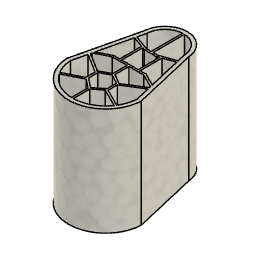
Molde fijo (Autodesk Fusion 360 design; units mm, degrees)
Autodesk Fusion 360 part; units mm, degrees
note: some values were not read from the file. Set by a fixed rule: which sketch regions a step uses.
sketch "Boceto1" plane through (0, 0, 0) normal (0, 0, 1) x (1, 0, 0)
  line L0 (0, -31.5) -> (3, -31.5) construction
  circle A0 centre (3, -22.5) radius 1.5 construction
  circle A1 centre (3, -10.5) radius 1.5 construction
  circle A2 centre (-5.5, -17.5) radius 1.5 construction
  line L1 (0, -35) -> (0, -31.5) construction
  line L2 (0, -35) -> (0, -5) construction
  line L3 (0, -20) -> (7.4517, -20) construction
  circle A3 centre (0, -16.5) radius 1.5 construction
  circle A4 centre (5.5, -17.5) radius 1.5 construction
  circle A5 centre (-3, -22.5) radius 1.5 construction
  circle A6 centre (-3, -10.5) radius 1.5 construction
  line L4 (0, -20) -> (-7.4517, -20) construction
  circle A7 centre (-5.5, -26.5) radius 1.5 construction
  line L5 (8.9851, -26.5171) -> (5.0484, -9.7858)
  arc A8 (-8.9851, -26.5171) -> (8.9851, -26.5171) centre (0, -26) ccw
  circle A9 centre (0, -26.5) radius 1.5 construction
  circle A10 centre (5.5, -26.5) radius 1.5 construction
  circle A11 centre (3, -31.5) radius 1.5 construction
  line L6 (0, -26.5) -> (5.5, -26.5) construction
  circle A12 centre (-3, -31.5) radius 1.5 construction
  line L7 (0, -35) -> (0, -26.5) construction
  line L8 (-5.0484, -9.7858) -> (-8.9851, -26.5171)
  arc A13 (5.0484, -9.7858) -> (-5.0484, -9.7858) centre (0, -10.0556) ccw
  arc A14 (6.0413, -9.6396) -> (-6.0413, -9.6396) centre (0, -10.0556) ccw
  line L9 (-6.0413, -9.6396) -> (-9.9909, -26.4257)
  arc A15 (-9.9909, -26.4257) -> (9.9909, -26.4257) centre (0, -26) ccw
  line L10 (9.9909, -26.4257) -> (6.0413, -9.6396)
  line L11 (5.5, -17.5) -> (4.5, -17.5) construction
  line L12 (-5.5, -17.5) -> (-4.5, -17.5) construction
  circle A16 centre (4.5, -17.5) radius 1.5 construction
  circle A17 centre (-4.5, -17.5) radius 1.5 construction
  line L13 (3, -10.5) -> (2.5, -10.5) construction
  line L14 (-3, -10.5) -> (-2.5, -10.5) construction
  circle A18 centre (2.5, -10.5) radius 1.5 construction
  circle A19 centre (-2.5, -10.5) radius 1.5 construction
  dimension "d3" = 0
  dimension "d4" = 9
  dimension "d7" = 0
  dimension "d8" = 10
  dimension "d11" = 0
  dimension "d12" = 21
  dimension "d15" = 0
  dimension "d16" = 9
  dimension "d17" = 3
  dimension "d18" = 3.5
  dimension "d19" = 3
  dimension "d20" = 3
  dimension "d21" = 3
  dimension "d22" = 5
  dimension "d23" = 5.5
  dimension "d24" = 1
  dimension "d48" = 1
  dimension "d49" = 1
  dimension "d50" = 3
  dimension "d51" = 3
  dimension "d52" = 0.5
  dimension "d53" = 3
  dimension "d54" = 3
  constraint midpoint L1.start A8
  constraint midpoint L2.end A13
  constraint midpoint L3.start L2
  constraint coincident L3.end L5
  constraint perpendicular L2 L3
  constraint coincident L4.end L8
  constraint perpendicular L2 L4
  constraint parallel L1 L2
  constraint perpendicular L0 L1
  constraint symmetric L2 A11 A12
  constraint coincident A9.centre L2
  constraint parallel L2 L7
  constraint perpendicular L6 L7
  constraint coincident A10.centre L6.end
  constraint symmetric L2 A7 A10
  constraint coincident A9.centre L6.start
  constraint coincident L0.end A11.centre
  constraint coincident A4.centre L11.start
  constraint horizontal L11
  constraint coincident A2.centre L12.start
  constraint horizontal L12
  constraint coincident L11.end A16.centre
  constraint coincident L12.end A17.centre
  constraint coincident A1.centre L13.start
  constraint perpendicular L2 L13
  constraint coincident A6.centre L14.start
  constraint perpendicular L2 L14
  constraint coincident L13.end A18.centre
  constraint coincident L14.end A19.centre
  measures "d17" diameter of A11
  measures "d18" distance of L1.start L0.start
  measures "d19" distance of L0.end L0.start
  measures "d20" diameter of A10
  measures "d21" diameter of A9
  measures "d22" distance of L0.start A9.centre
  measures "d23" distance of A9.centre A10.centre
  measures "d48" distance of A4.centre L11.end
  measures "d49" distance of A2.centre L12.end
  measures "d50" diameter of A16
  measures "d51" diameter of A17
  measures "d52" distance of A1.centre L13.end
  measures "d53" diameter of A18
  measures "d54" diameter of A19
extrude "Extruir1" add sketch "Boceto1" along normal blind 29
sketch "Boceto2" plane through (0, 0, 29) normal (0, 0, 1) x (-1, 0, 0)
  arc A0 (-5.0484, 9.7858) -> (5.0484, 9.7858) centre (0, 10.0556) ccw
  line L0 (-5.0484, 9.7858) -> (-8.9851, 26.5171)
  arc A1 (8.9851, 26.5171) -> (-8.9851, 26.5171) centre (0, 26) ccw
  line L1 (8.9851, 26.5171) -> (5.0484, 9.7858)
  line L2 (-9.9909, 26.4257) -> (-6.0413, 9.6396)
  arc A2 (-6.0413, 9.6396) -> (6.0413, 9.6396) centre (0, 10.0556) ccw
  line L3 (6.0413, 9.6396) -> (9.9909, 26.4257)
  arc A3 (9.9909, 26.4257) -> (-9.9909, 26.4257) centre (0, 26) ccw
  circle A4 centre (-5.5, 26.5) radius 1.5
  circle A5 centre (-3, 31.5) radius 1.5
  circle A6 centre (3, 31.5) radius 1.5
  circle A7 centre (0, 26.5) radius 1.5
  line L4 (0, 35) -> (0, 26.5)
  circle A8 centre (-3, 22.5) radius 1.5
  circle A9 centre (-5.5, 17.5) radius 1.5
  circle A10 centre (-3, 10.5) radius 1.5
  circle A11 centre (3, 10.5) radius 1.5
  circle A12 centre (0, 16.5) radius 1.5
  circle A13 centre (5.5, 17.5) radius 1.5
  circle A14 centre (3, 22.5) radius 1.5
  circle A15 centre (5.5, 26.5) radius 1.5
  line L5 (-3, 31.5) -> (-5.5, 26.5) construction
  line L6 (3, 31.5) -> (5.5, 26.5) construction
  line L7 (-3, 22.5) -> (0, 26.5) construction
  line L8 (-3, 22.5) -> (-5.5, 26.5) construction
  line L9 (-5.5, 17.5) -> (-3, 22.5) construction
  line L10 (-5.5, 17.5) -> (0, 16.5) construction
  line L11 (0, 16.5) -> (-3, 10.5) construction
  line L12 (-4.25, 29) -> (-7.6694, 30.7097)
  line L13 (-4.25, 24.5) -> (-7.9643, 22.1786)
  line L14 (-4.25, 20) -> (-7.8786, 21.8143)
  line L15 (-3, 28.375) -> (2.011, 25.8695) construction
  line L16 (-3, 25.2812) -> (3.382, 29.27) construction
  line L17 (-3, 26.5) -> (-3, 28.375)
  line L18 (0, 23.6397) -> (-3, 25.3603)
  line L19 (0, 30.75) -> (-3, 28.375)
  line L20 (-4.25, 29) -> (-3, 28.375)
  line L21 (-4.25, 24.5) -> (-2.9341, 25.3225)
  line L22 (-4.25, 20) -> (0, 20)
  line L23 (-1.5, 13.5) -> (0, 13.5)
  line L24 (-1.5, 13.5) -> (-5.5795, 12.043)
  line L25 (0, 30.75) -> (3, 28.375)
  line L26 (4.25, 29) -> (7.6694, 30.7097)
  line L27 (4.25, 29) -> (3, 28.375)
  line L28 (3, 26.5) -> (3, 28.375)
  line L29 (3, 25.3603) -> (3, 25.2812)
  line L30 (0, 23.6397) -> (3, 25.3603)
  line L31 (4.25, 24.5) -> (2.9341, 25.3225)
  line L32 (4.25, 24.5) -> (7.9643, 22.1786)
  line L33 (4.25, 20) -> (7.8786, 21.8143)
  line L34 (4.25, 20) -> (0, 20)
  line L35 (1.5, 13.5) -> (5.5795, 12.043)
  line L36 (1.5, 13.5) -> (0, 13.5)
  line L37 (-1.5866, 14) -> (-5.7476, 12.5139)
  line L38 (-1.5866, 14) -> (0, 14)
  line L39 (-4.368, 19.5) -> (0, 19.5)
  line L40 (-4.368, 19.5) -> (-8.1022, 21.3671)
  line L41 (-3, 26.5) -> (-3, 25.3603)
  line L42 (3, 26.5) -> (3, 25.3603)
  line L43 (0, 30.1123) -> (-2.5, 28.1331)
  line L44 (-2.5, 26.5) -> (-2.5, 28.1331)
  line L45 (-2.5, 26.5) -> (-2.5, 25.6499)
  line L46 (0, 24.2161) -> (-2.5, 25.6499)
  line L47 (0, 24.2161) -> (2.5, 25.6499)
  line L48 (2.5, 26.5) -> (2.5, 25.6499)
  line L49 (2.5, 26.5) -> (2.5, 28.1331)
  line L50 (0, 30.1123) -> (2.5, 28.1331)
  line L51 (-4.515, 24.924) -> (-8.2293, 22.6026)
  line L52 (-4.515, 24.924) -> (-3, 25.8709)
  line L53 (4.515, 24.924) -> (3, 25.8709)
  line L54 (4.515, 24.924) -> (8.2293, 22.6026)
  line L55 (-4.0264, 29.4472) -> (-7.4457, 31.1569)
  line L56 (-4.0264, 29.4472) -> (-2.5672, 28.7176)
  line L57 (3, 28.934) -> (7.4457, 31.1569)
  line L58 (4.0264, 29.4472) -> (2.5672, 28.7176)
  line L59 (2.8037, 19.5) -> (2.7874, 19.5894)
  line L60 (4.368, 19.5) -> (8.1022, 21.3671)
  line L61 (4.368, 19.5) -> (0, 19.5)
  line L62 (1.5866, 14) -> (0, 14)
  line L63 (1.5866, 14) -> (5.7476, 12.5139)
  line L64 (0, 5) -> (0, 13.5)
  line L65 (0.25, 5) -> (0.25, 13.5)
  line L66 (-0.25, 5) -> (-0.25, 13.5)
  line L67 (-0.25, 23.7831) -> (-0.25, 20)
  line L68 (0.25, 23.7831) -> (0.25, 20)
  line L69 (-0.25, 35) -> (-0.25, 30.5521)
  line L70 (0.25, 35) -> (0.25, 30.5521)
  line L71 (0, 26.5) -> (0, 25)
  line L72 (0, 20) -> (0, 19.5)
  line L73 (0, 18) -> (0, 16.5)
  line L74 (-3.2659, 16.9578) -> (-3.2419, 17.0894)
  line L75 (-2.75, 17) -> (-2.75, 19.5)
  line L76 (-2.75, 17) -> (-2.75, 13.5845)
  line L77 (-2.75, 19.5) -> (-2.25, 19.5)
  line L78 (-2.25, 19.5) -> (-2.25, 13.7631)
  line L79 (2.25, 19.5) -> (2.25, 13.7631)
  line L80 (2.75, 17) -> (2.75, 13.5845)
  line L81 (2.75, 17) -> (2.75, 19.5)
  dimension "d27" = 7
  dimension "d28" = 9
  dimension "d29" = -0.5
  dimension "d31" = 0.5
  dimension "d32" = -0.5
  dimension "d38" = 0.5
  dimension "d39" = -0.5
  dimension "d40" = 0.25
  dimension "d41" = -0.25
  dimension "d55" = 0.5
  constraint coincident A5.centre L5.start
  constraint coincident A4.centre L5.end
  constraint coincident A6.centre L6.start
  constraint coincident A15.centre L6.end
  constraint coincident A8.centre L7.start
  constraint coincident A7.centre L4.end
  constraint coincident A9.centre L9.start
  constraint coincident A12.centre L10.end
  constraint coincident A10.centre L11.end
  constraint midpoint L5 L12.start
  constraint coincident A1 L12.end
  constraint perpendicular L5 L12
  constraint midpoint L8 L13.start
  constraint coincident L0 L13.end
  constraint perpendicular L8 L13
  constraint midpoint L9 L14.start
  constraint coincident L0 L14.end
  constraint perpendicular L9 L14
  constraint midpoint A0 L64.start
  constraint perpendicular L5 L15
  constraint perpendicular L8 L16
  constraint vertical L17
  constraint midpoint L4 L19.start
  constraint perpendicular L5 L20
  constraint perpendicular L8 L21
  constraint coincident L22.end L71
  constraint perpendicular L22 L71
  constraint midpoint L10 L75.start
  constraint midpoint L11 L23.start
  constraint coincident L0 L24.end
  constraint symmetric L12.start L26.start L71
  constraint symmetric L12.end L26.end L71
  constraint symmetric L13.start L31.start L71
  constraint symmetric L13.end L32.end L71
  constraint symmetric L14.start L33.start L71
  constraint symmetric L14.end L33.end L71
  constraint symmetric L17.start L28.start L71
  constraint symmetric L15.start L25.end L71
  constraint symmetric L16.start L29.end L71
  constraint symmetric L18.end L29.start L71
  constraint symmetric L19.start L25.start L71
  constraint symmetric L22.end L34.end L71
  constraint symmetric L23.start L35.start L71
  constraint symmetric L23.end L36.end L71
  constraint symmetric L24.end L35.end L71
  constraint parallel L17 L41
  constraint coincident L18 L21.end
  constraint coincident L16.start L21
  constraint coincident L30 L31.end
  constraint coincident L29.end L31
  constraint coincident L19 L56.end
  constraint coincident L58.start L57
  constraint coincident L25 L58.end
  constraint perpendicular L23 L64
  constraint coincident L18 L67.start
  constraint coincident L30 L68.start
  constraint coincident L25 L70.end
  constraint coincident L19 L69.end
  constraint coincident A7 L71.end
  constraint coincident A12 L73.start
  constraint collinear L72 L73
  constraint coincident L10 L74.end
  constraint coincident L39 L75.end
  constraint perpendicular L39 L75
  constraint coincident L37 L76.end
  constraint parallel L75 L76
  constraint perpendicular L75 L77
  constraint coincident L37 L78.end
  constraint perpendicular L39 L78
  constraint coincident L61 L59.start
  constraint symmetric L75.start L73 L80.start
  constraint symmetric L73 L75.end L81.end
  constraint symmetric L73 L76.end L80.end
  constraint symmetric L73 L77.end L79.start
  constraint symmetric L73 L78.end L79.end
  measures "d27" distance of L12.start L15.end
  measures "d28" distance of L13.start L16.end
  measures "d55" distance of L75.end L77.end
extrude "Extruir2" add sketch "Boceto2" against normal blind 23.5 contours A0 L23 L64 L66 | L0 L1 L23 L24 L35 L36 L37 L38 L62 L63 | A0 L36 L64 L65 | L37 L39 L75 L76 L77 L78 | L0 L14 L22 L39 L40 L72 L77 | L1 L33 L34 L60 L61 L72 | L61 L63 L79 L80 L81 | L0 L13 L18 L21 L41 L51 L52 | L18 L22 L30 L34 L67 L68 | L17 L18 L19 L25 L28 L30 L41 L42 | A1 L12 L19 L20 L55 L56 | L1 L29 L31 L32 L42 L53 L54 | A1 L4 L19 L69 | A1 L4 L25 L70 | A1 L25 L26 L27 L57 L58
equation "d25 = 5 mm + 18 mm + 5 mm + 1 mm"
